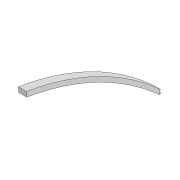
# Autodesk Inventor part: Part_11_p1
Saved by Autodesk Inventor 2022 (Build 260153000, 153)
## iProperties
Created: 2022-04-24
Part Number: Part_11_p1
Material: Generic
Document SubType Name: Modeling
Designer: dell
Density: 1 g/cm^3
Appearance: Default
Author: dell
Autodesk Inventor part; units mm, degrees
ref_plane "YZ Plane" through (0, 0, 0) normal (1, 0, 0) x (0, 1, 0)
ref_plane "XZ Plane" through (0, 0, 0) normal (0, 1, 0) x (-1, 0, 0)
ref_plane "XY Plane" through (0, 0, 0) normal (0, 0, 1) x (1, 0, 0)
sketch "Sketch1" plane through (0, 0, 0) normal (0, 1, 0) x (-1, 0, 0)
  line L0 (0, 0) -> (0, -160) construction
  line L1 (5, 0) -> (5, -160)
  line L2 (-5, -160) -> (-5, 0)
  arc A0 (5, 0) -> (-5, 0) centre (0, 0) ccw
  arc A1 (-5, -160) -> (5, -160) centre (0, -160) ccw
  circle A2 centre (0, 0) radius 1.65
  line L3 (0, -30) -> (0, -120) construction
  line L4 (1.65, -30) -> (1.65, -120)
  line L5 (-1.65, -120) -> (-1.65, -30)
  arc A3 (1.65, -30) -> (-1.65, -30) centre (0, -30) ccw
  arc A4 (-1.65, -120) -> (1.65, -120) centre (0, -120) ccw
  point P0 (0, -80)
  point P1 (0, -75)
  dimension "d0" = 160
  dimension "d1" = 10
  dimension "d2" = 3.3
  dimension "d3" = 30
  dimension "d5" = 120
  dimension "d6" = 3.3
  constraints: 16 end point, 8 point on circle, 8 tangent, 5 centre point, 2 midpoint, 2 parallel, 2 point on line, 1 coincident, 1 vertical
  measures "d0" distance of L0.end L0.start
  measures "d1" distance between parallel lines of L1 L2
  measures "d2" diameter of A2
  measures "d3" distance of L0.start L3.start
  measures "d5" distance of L0.start L3.end
  measures "d6" distance between parallel lines of L5 L4
extrude "Extrusion1" add sketch "Sketch1" along normal blind 6
sketch "Sketch2" plane through (5, 0, 0) normal (1, 0, 0) x (0, 0, -1)
  line L0 (160, 0) -> (160, 6) projected
  line L1 (0, 0) -> (160, 0) projected
  line L2 (160, 0) -> (160, 6) projected
  line L3 (0, 6) -> (160, 6) projected
  line L4 (0, 0) -> (0, 6) projected
  line L5 (160, 0) -> (160, 0) projected
  line L6 (160, 0) -> (160, 6) projected
  line L7 (160, 6) -> (160, 6) projected
  line L8 (160, 0) -> (160, 6) projected
  line L9 (160, 0) -> (0, 0) projected
  arc A0 (373.775, -84) -> (160, 0) centre (160, -314.0223) ccw
  line L10 (160, 6) -> (0, 6) projected
  arc A1 (373.775, -78) -> (160, 6) centre (160, -308.0223) ccw
  line L11 (373.775, -78) -> (373.775, -84)
  line L12 (0, 0) -> (160, 0) projected
  dimension "d9" = 6
  dimension "d10" = 373.775
  dimension "d11" = 90
  constraints: 4 point on circle, 2 centre point, 2 end point, 2 tangent, 1 vertical
  measures "d9" distance of L11.start L11.end
  measures "d10" distance between parallel lines of L4 L11
  measures "d11" distance from line of L3 L11.end
extrude "Extrusion2" add sketch "Sketch2" against normal blind 10 contours L0 A1 L11 A0
fillet "Fillet1" radius 2 4 edges at (0, -78, -373.775) (5, -81, -373.775) (-5, -81, -373.775) (0, -84, -373.775)
sketch "Sketch3" plane through (0, 6, 0) normal (0, 1, 0) x (1, 0, 0)
  line L0 (36.6774, -16.9321) -> (-64.8889, -16.9321)
  line L1 (-64.8889, -16.9321) -> (-64.8889, 211.3912)
  line L2 (-64.8889, 211.3912) -> (36.6774, 211.3912)
  line L3 (36.6774, 211.3912) -> (36.6774, -16.9321)
  line L4 (-92.1247, 397.3107) -> (101.238, 397.3107)
  line L5 (101.238, 397.3107) -> (101.238, -55.9315)
  line L6 (101.238, -55.9315) -> (-92.1247, -55.9315)
  line L7 (-92.1247, -55.9315) -> (-92.1247, 397.3107)
  point P0 (0, 0)
  constraints: 16 end point, 4 parallel, 2 horizontal, 2 perpendicular
extrude "Extrusion3" cut sketch "Sketch3" against normal blind 100 contours L0 L1 L2 L3
body "Solid1"
